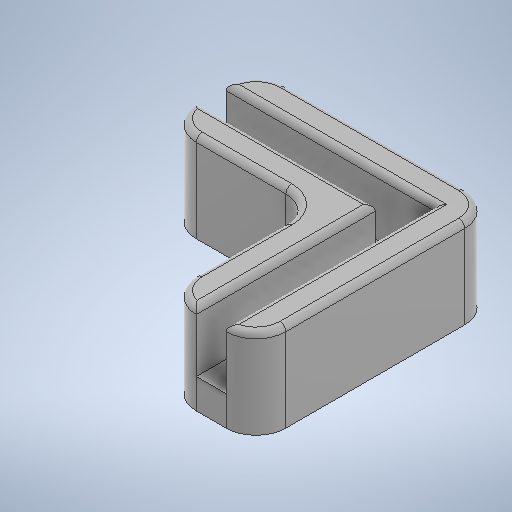
# Autodesk Inventor part: TSU_Corner_Top_Clamp
Saved by Autodesk Inventor 2025.2 (Build 292293000, 293)
## iProperties
Created: 2025-01-07
Part Number: TSU_Corner_Top_Clamp
Material: Generic
Document SubType Name: Modeling
Designer: Matt Tidd
Density: 1 g/cm^3
Appearance: Default
Author: Matt Tidd
Autodesk Inventor part; units mm, degrees
ref_plane "YZ Plane" through (0, 0, 0) normal (1, 0, 0) x (0, 1, 0)
ref_plane "XZ Plane" through (0, 0, 0) normal (0, 1, 0) x (-1, 0, 0)
ref_plane "XY Plane" through (0, 0, 0) normal (0, 0, 1) x (1, 0, 0)
sketch "Sketch1" plane through (0, 0, 0) normal (0, 1, 0) x (-1, 0, 0)
  line L0 (0, 0) -> (30, 0)
  line L1 (30, 0) -> (30, -80)
  line L2 (30, -80) -> (0, -80)
  line L3 (0, -80) -> (0, 0)
  line L4 (30, -80) -> (80, -80)
  line L5 (80, -80) -> (80, -50)
  line L6 (80, -50) -> (30, -50)
  line L7 (30, -50) -> (30, -80)
  dimension "d0" = 30
  dimension "d1" = 80
  dimension "d2" = 50
  dimension "d3" = 30
  constraints: 16 end point, 4 parallel, 2 horizontal, 2 perpendicular
  measures "d0" distance of L1.end L2.end
  measures "d1" distance of L0.end L1.end
  measures "d2" distance of L6.end L5.end
  measures "d3" distance of L5.end L4.end
extrude "Extrusion1" add sketch "Sketch1" along normal blind 10
sketch "Sketch2" plane through (0, 10, 0) normal (0, 1, 0) x (1, 0, 0)
  line L0 (-30, 0) -> (0, 0) projected
  line L1 (-30, 0) -> (-20, 0)
  line L2 (-20, 0) -> (-20, 50)
  line L3 (-20, 50) -> (-30, 50)
  line L4 (-30, 50) -> (-30, 0)
  line L5 (-80, 80) -> (-80, 50) projected
  line L6 (-80, 50) -> (-20, 50)
  line L7 (-20, 50) -> (-20, 60)
  line L8 (-20, 60) -> (-80, 60)
  line L9 (-80, 60) -> (-80, 50)
  line L10 (-80, 80) -> (0, 80)
  line L11 (0, 80) -> (0, 70)
  line L12 (0, 70) -> (-80, 70)
  line L13 (-80, 70) -> (-80, 80)
  line L14 (0, 70) -> (-10, 70)
  line L15 (-10, 70) -> (-10, 0)
  line L16 (-10, 0) -> (0, 0)
  line L17 (0, 0) -> (0, 70)
  dimension "d6" = 10
  dimension "d7" = 10
  dimension "d8" = 80
  dimension "d9" = 10
  dimension "d10" = 10
  constraints: 32 end point, 8 parallel, 4 horizontal, 4 perpendicular, 2 point on line
  measures "d6" distance of L3.end L2.end
  measures "d7" distance of L7.end L6.end
  measures "d8" distance of L11.end L12.end
  measures "d9" distance of L10.end L11.end
  measures "d10" distance of L16.end L15.end
extrude "Extrusion2" add sketch "Sketch2" along normal blind 20 contours L4 L3 L2 L0 | L6 L5 L8 L7 L3 | L15 L12 L17 L0 | L12 L5 L10 L11
fillet "Fillet1" radius 10 6 edges at (-30, 15, -50) (-30, 15, 0) (-80, 15, -50) (-80, 15, -80) (0, 15, -80) (0, 15, 0)
fillet "Fillet2" radius 2 12 edges at (-55, 30, -50) (-77.0711, 30, -52.9289) (-30, 30, -25) (-27.0711, 30, -2.9289) (-77.0711, 30, -77.0711) (-2.9289, 30, -77.0711) (-2.9289, 30, -2.9289) (-40, 30, -80) (-45, 30, -70) (-50, 30, -60) (-10, 30, -35) (-20, 30, -30)
body "Solid1"
